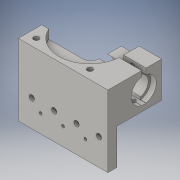
# Autodesk Inventor part: Galvomount-22mm-diameter-Left-Scanlab-V4
Saved by Autodesk Inventor 2016 (Build 200138000, 138)
## iProperties
Created: 2016-08-10
Part Number: Galvomount-22mm-diameter-Left-Scanlab-V4
Material: Generic
Document SubType Name: Modeling
Designer: voigt
Density: 1 g/cm^3
Appearance: Default
Author: voigt
Autodesk Inventor part; units mm, degrees
ref_plane "YZ Plane" through (0, 0, 0) normal (1, 0, 0) x (0, 1, 0)
ref_plane "XZ Plane" through (0, 0, 0) normal (0, 1, 0) x (-1, 0, 0)
ref_plane "XY Plane" through (0, 0, 0) normal (0, 0, 1) x (1, 0, 0)
sketch "Sketch1" plane through (0, 0, 0) normal (0, 0, 1) x (1, 0, 0)
  line L0 (0, 32) -> (0, -52) construction
  line L1 (-60, 0) -> (80, 0) construction
  line L2 (-40, 20) -> (60, 20)
  line L3 (60, 20) -> (60, -40)
  line L4 (60, -40) -> (-40, -40)
  line L5 (-40, -40) -> (-40, 20)
  point P0 (0, 0)
  dimension "d0" = 20
  dimension "d1" = 40
  dimension "d2" = 40
  dimension "d3" = 60
  constraints: 8 end point, 2 parallel, 1 horizontal, 1 perpendicular
  measures "d0" distance between parallel lines of L1 L2
  measures "d1" distance between parallel lines of L4 L1
  measures "d2" distance between parallel lines of L5 L0
  measures "d3" distance between parallel lines of L0 L3
extrude "Extrusion1" add sketch "Sketch1" against normal blind 40
sketch "Sketch2" plane through (0, 0, 0) normal (0, 0, 1) x (1, 0, 0)
  line L0 (-40, 20) -> (60, 20) construction
  line L1 (-40, -40) -> (-40, 20) construction
  line L2 (60, -40) -> (-40, -40) construction
  line L3 (60, 20) -> (60, -40) construction
  line L4 (0, 98) -> (0, -63) construction
  line L5 (-60, 0) -> (80, 0) construction
  line L6 (0, 40) -> (0, 0) construction
  line L7 (-40, 20) -> (60, 20) projected
  line L8 (-35, 40) -> (-35, 0)
  line L9 (35, 0) -> (35, 40)
  arc A0 (35, 40) -> (-35, 40) centre (0, 40) ccw
  arc A1 (-35, 0) -> (35, 0) centre (0, 0) ccw
  point P0 (0, 20)
  dimension "d6" = 70
  constraints: 8 end point, 4 point on circle, 4 tangent, 2 centre point, 2 point on line, 1 midpoint, 1 parallel, 1 perpendicular
  measures "d6" diameter of A1
extrude "Extrusion2" cut sketch "Sketch2" against normal blind 10
sketch "Sketch3" plane through (60, -40, 0) normal (1, 0, 0) x (0, 0, -1)
  line L0 (0, 60) -> (0, 0) construction
  line L1 (0, 0) -> (40, 0) construction
  line L2 (40, 60) -> (40, 0) construction
  line L3 (0, 60) -> (40, 60) construction
  line L4 (0, 40) -> (40, 40) construction
  line L5 (40, 0) -> (40, 60) construction
  line L6 (0, 60) -> (40, 60) construction
  line L7 (20, 60) -> (20, 0) construction
  circle A0 centre (20, 40) radius 11
  dimension "d9" = 22
  constraints: 4 end point, 3 midpoint, 2 point on line, 1 centre point, 1 perpendicular
  measures "d9" diameter of A0
extrude "Extrusion3" cut sketch "Sketch3" against normal up to next
sketch "Sketch6" plane through (0, 0, 0) normal (0, 0, 1) x (1, 0, 0)
  line L0 (0, 44) -> (0, -54) construction
  line L1 (-60, 0) -> (80, 0) construction
  line L2 (-30, 30) -> (30, 30) construction
  line L3 (30, 30) -> (30, -30) construction
  line L4 (30, -30) -> (-30, -30) construction
  line L5 (-30, -30) -> (-30, 30) construction
  point P0 (0, 0)
  dimension "d19" = 60
  dimension "d20" = 60
  constraints: 8 end point, 2 coincident, 2 parallel, 1 horizontal, 1 perpendicular, 2 other
  measures "d19" distance of L2.start L2.end
  measures "d20" distance of L4.end L2.start
hole "Hole1" at (-30, -30, 0) at (30, -30, 0) direction (0, 0, -1) diameter 6 depth 30 tip angle 118
sketch "Sketch16" plane through (-40, -40, 0) normal (-1, 0, 0) x (0, 0, 1)
  line L0 (-40, 0) -> (-40, 60) construction
  line L1 (0, 0) -> (-40, 0) construction
  line L2 (0, 0) -> (0, 60) construction
  line L3 (0, 13) -> (0, 7) construction
  line L4 (-30, 7) -> (-30, 13) construction
  line L5 (-30, 10) -> (0, 10) construction
  circle A0 centre (-20, 40) radius 11 projected
  line L6 (0, 60) -> (-40, 60) projected
  point P0 (0, 40)
  point P1 (-10, 10)
  dimension "d86" = 10
  constraints: 2 end point, 2 midpoint, 1 point on line
  measures "d86" distance from line of L2 point (-10, 10)
hole "Hole7" at (-40, -30, -10) direction (1, 0, 0) diameter 2.156 depth 8.865 tip angle 118 thread size "4-40 UNC" class "2B" standard "ANSI Unified Screw Threads"
sketch "Sketch18" plane through (-40, -40, 0) normal (-1, 0, 0) x (0, 0, 1)
  circle A0 centre (-10, 10) radius 1.078 projected
  line L0 (-40, 0) -> (-40, 60) projected
  line L1 (0, 0) -> (-40, 0) projected
  line L2 (0, 0) -> (0, 60) projected
  circle A1 centre (-20, 40) radius 11 projected
  line L3 (0, 60) -> (-40, 60) projected
  point P0 (0, 40)
extrude "Extrusion10" cut sketch "Sketch18" against normal blind 5 contours A1
sketch "Sketch19" plane through (60, -40, 0) normal (1, 0, 0) x (0, 0, -1)
  line L0 (0, 60) -> (40, 60) projected
  line L1 (0, 60) -> (0, 0) projected
  line L2 (0, 0) -> (40, 0) projected
  line L3 (40, 60) -> (40, 0) projected
  circle A0 centre (20, 40) radius 11 projected
  point P0 (0, 40)
extrude "Extrusion11" cut sketch "Sketch19" against normal blind 6 contours A0
sketch "Sketch23" plane through (60, -40, 0) normal (1, 0, 0) x (0, 0, -1)
  circle A0 centre (20, 40) radius 11 construction
  line L0 (0, 60) -> (0, 0) construction
  line L1 (0, 0) -> (40, 0) construction
  line L2 (40, 60) -> (40, 0) construction
  line L3 (0, 60) -> (40, 60) construction
  line L4 (0, 42.5) -> (34, 42.5)
  line L5 (34, 42.5) -> (34, 37.5)
  line L6 (34, 37.5) -> (0, 37.5)
  line L7 (0, 37.5) -> (0, 42.5)
  line L8 (0, 40) -> (20, 40) construction
  dimension "d119" = 5
  dimension "d120" = 14
  constraints: 10 end point, 2 horizontal, 2 parallel, 1 perpendicular, 1 point on line, 1 other
  measures "d119" distance between parallel lines of L6 L4
  measures "d120" distance from line of L8.end L5
extrude "Extrusion15" cut sketch "Sketch23" against normal up to next
sketch "Sketch24" plane through (-40, 20, -40) normal (0, 1, 0) x (1, 0, 0)
  line L0 (75, -30) -> (75, -40) construction
  line L1 (75, -40) -> (100, -40) construction
  line L2 (100, -40) -> (100, 0) construction
  line L3 (0, 0) -> (100, 0) construction
  line L4 (0, -40) -> (0, 0) construction
  line L5 (0, -40) -> (5, -40) construction
  line L6 (5, -40) -> (5, -30) construction
  line L7 (5, -30) -> (75, -30) construction
  line L8 (100, -6) -> (0, -6) construction
  line L9 (100, -6) -> (0, -6) projected
  line L10 (0, -40) -> (55, -40)
  line L11 (55, -40) -> (55, -6)
  line L12 (55, -6) -> (0, -6)
  line L13 (0, -6) -> (0, -40)
  line L14 (40, -40) -> (40, 0) construction
  line L15 (0, 0) -> (100, 0) construction
  dimension "d123" = 15
  constraints: 10 end point, 2 parallel, 2 perpendicular, 2 point on line, 1 horizontal
  measures "d123" distance between parallel lines of L14 L11
extrude "Extrusion16" cut sketch "Sketch24" against normal blind 34
fillet "Fillet3" radius 10 1 edges at (15, -14, -22)
sketch "Sketch25" plane through (0, 0, -40) normal (0, 0, -1) x (-1, 0, 0)
  line L0 (40, 20) -> (-60, 20) construction
  line L1 (-60, 20) -> (-60, -40) construction
  line L2 (-60, -40) -> (40, -40) construction
  line L3 (40, -40) -> (40, 20) construction
  line L4 (-60, 20) -> (-60, -40) projected
  line L5 (40, -28.922) -> (40, -31.078) projected
  line L6 (-60, -40) -> (40, -40)
  line L7 (40, -40) -> (40, -30)
  line L8 (40, -30) -> (-60, -30)
  line L9 (-60, -30) -> (-60, -40)
  point P0 (0, 0)
  dimension "d127" = 10
  constraints: 8 end point, 2 parallel, 1 horizontal, 1 midpoint, 1 perpendicular
  measures "d127" distance of L7.end L6.end
extrude "Extrusion17" add sketch "Sketch25" along normal blind 40
sketch "Sketch26" plane through (-40, 20, -40) normal (0, 1, 0) x (1, 0, 0)
  line L0 (100, 40) -> (0, 40) construction
  line L1 (55, -6) -> (55, -30) construction
  line L2 (55, -30) -> (75, -30) construction
  line L3 (75, -30) -> (75, -40) construction
  line L4 (75, -40) -> (100, -40) construction
  line L5 (100, -40) -> (100, 0) construction
  line L6 (0, 0) -> (100, 0) construction
  line L7 (0, -6) -> (0, 0) construction
  line L8 (0, -6) -> (55, -6) construction
  line L9 (0, -6) -> (55, -6) projected
  line L10 (0, 0) -> (100, 0) projected
  line L11 (0, -6) -> (55, -6)
  line L12 (55, -6) -> (55, 0)
  line L13 (55, 0) -> (0, 0)
  line L14 (0, 0) -> (0, -6)
  line L15 (55, -6) -> (55, -30) projected
  point P0 (40, -40)
  constraints: 8 end point, 2 parallel, 1 collinear, 1 horizontal, 1 perpendicular, 1 point on line
extrude "Extrusion18" cut sketch "Sketch26" against normal blind 10
sketch "Sketch27" plane through (-40, -30, -40) normal (0, 1, 0) x (1, 0, 0)
  line L0 (100, 0) -> (0, 0) construction
  line L1 (100, 0) -> (100, 40) construction
  line L2 (0, 40) -> (100, 40) construction
  line L3 (0, 0) -> (0, 40) construction
  line L4 (0, -40) -> (0, 40) construction
  line L5 (0, 10) -> (100, 10) construction
  line L6 (40, -40) -> (40, 40) construction
  line L7 (0, 40) -> (100, 40) construction
  point P0 (40, 10)
  point P1 (15, 10)
  point P2 (65, 10)
  point P3 (90, 10)
  dimension "d132" = 10
  dimension "d154" = 25
  dimension "d155" = 25
  dimension "d156" = 25
  constraints: 8 point on line, 4 end point, 1 perpendicular, 1 vertical
  measures "d132" distance between parallel lines of L0 L5
  measures "d154" distance of point (15, 10) point (40, 10)
  measures "d155" distance of point (65, 10) point (40, 10)
  measures "d156" distance of point (65, 10) point (90, 10)
sketch "Sketch28" plane through (60, 20, 0) normal (1, 0, 0) x (0, 0, -1)
  line L0 (34, -22.5) -> (30.7121, -22.5) construction
  arc A0 (9.2879, -22.5) -> (30.7121, -22.5) centre (20, -20) ccw construction
  line L1 (9.2879, -22.5) -> (0, -22.5) construction
  line L2 (0, -22.5) -> (0, -60) construction
  line L3 (0, -60) -> (80, -60) construction
  line L4 (80, -50) -> (80, -60) construction
  line L5 (40, -50) -> (80, -50) construction
  line L6 (40, 0) -> (40, -50) construction
  line L7 (0, 0) -> (40, 0) construction
  line L8 (0, 0) -> (0, -17.5) construction
  line L9 (0, -17.5) -> (9.2879, -17.5) construction
  arc A1 (30.7121, -17.5) -> (9.2879, -17.5) centre (20, -20) ccw construction
  line L10 (30.7121, -17.5) -> (34, -17.5) construction
  line L11 (34, -17.5) -> (34, -22.5) construction
  circle A2 centre (20, -20) radius 14
  point P0 (0, -20)
  dimension "d133" = 28
  constraints: 1 centre point, 1 coincident
  measures "d133" diameter of A2
extrude "Extrusion19" cut sketch "Sketch28" against normal blind 6
sketch "Sketch29" plane through (60, 20, 0) normal (0, 1, 0) x (1, 0, 0)
  line L0 (-6, 6.225) -> (-6, 9.2879) construction
  line L1 (-25.0894, 9.2879) -> (-6, 9.2879) construction
  line L2 (-25.0894, 0) -> (-25.0894, 9.2879) construction
  line L3 (0, 0) -> (-25.0894, 0) construction
  line L4 (0, 6.225) -> (0, 0) construction
  line L5 (0, 6.225) -> (-6, 6.225) construction
  line L6 (-45, 40) -> (-45, 10) construction
  line L7 (-45, 10) -> (-25, 10) construction
  line L8 (-25, 10) -> (-25, 0) construction
  line L9 (-25, 0) -> (0, 0) construction
  line L10 (0, 0) -> (0, 40) construction
  line L11 (-45, 40) -> (0, 40) construction
  point P0 (-60, 0)
  point P1 (-15, 5)
  dimension "d136" = 5
  dimension "d138" = 10
  measures "d136" distance from line of L3 point (-15, 5)
  measures "d138" distance from line of L8 point (-15, 5)
hole "Hole9" at (45, 20, -5) direction (0, -1, 0) diameter 5 end up to surface counterbore diameter 9 counterbore depth 5
sketch "Sketch30" plane through (34.9106, -2.5, 0) normal (0, 1, 0) x (1, 0, 0)
  circle A0 centre (10.0894, 5) radius 4.5 construction
  circle A1 centre (10.0894, 5) radius 2.5 construction
  point P0 (-34.9106, 0)
  constraints: 1 coincident
hole "Hole10" at (45, -2.5, -5) direction (0, -1, 0) diameter 4.134 depth 14.2 tip angle 118 thread size "M5x0.8" class "6H" standard "ISO Metric profile"
hole "Hole11" at (0, -30, -50) at (-25, -30, -50) at (25, -30, -50) at (50, -30, -50) direction (0, -1, 0) diameter 6 end through all counterbore diameter 10.5 counterbore depth 6.5
sketch "Sketch31" plane through (0, 0, -40) normal (0, 0, -1) x (-1, 0, 0)
  line L0 (-15, 10) -> (-15, 20) construction
  line L1 (-15, 20) -> (-60, 20) construction
  line L2 (-60, 20) -> (-60, -30) construction
  line L3 (-60, -30) -> (40, -30) construction
  line L4 (40, -30) -> (40, 10) construction
  line L5 (40, 10) -> (-15, 10) construction
  line L6 (-60, -10) -> (40, -10) construction
  point P0 (0, 0)
  point P1 (-35, -10)
  point P2 (15, -10)
  point P3 (-10, -10)
  dimension "d164" = 20
  dimension "d165" = 25
  dimension "d166" = 25
  constraints: 3 point on line, 2 end point, 2 midpoint, 1 perpendicular
  measures "d164" distance between parallel lines of L5 L6
  measures "d165" distance of point (-10, -10) point (15, -10)
  measures "d166" distance of point (-10, -10) point (-35, -10)
hole "Hole12" at (35, -10, -40) at (-15, -10, -40) at (10, -10, -40) direction (0, 0, 1) diameter 3.242 depth 10 tip angle 118 thread size "M4x0.7" class "6H" standard "ANSI Metric M Profile"
sketch "Sketch32" plane through (-40, -30, -40) normal (0, 1, 0) x (1, 0, 0)
  circle A0 centre (65, 10) radius 5.25 construction
  circle A1 centre (40, 10) radius 5.25 construction
  circle A2 centre (15, 10) radius 5.25 construction
  circle A3 centre (90, 10) radius 5.25 construction
  line L0 (100, 0) -> (0, 0) construction
  line L1 (100, 0) -> (100, 40) construction
  line L2 (0, 40) -> (100, 40) construction
  line L3 (0, 0) -> (0, 40) construction
  line L4 (100, 0) -> (100, 40) construction
  line L5 (100, 20) -> (0, 20) construction
  line L6 (0, 0) -> (0, 40) construction
  point P0 (40, -40)
  point P1 (50, 20)
  point P2 (25, 20)
  point P3 (75, 20)
  dimension "d174" = 50
  dimension "d175" = 25
  dimension "d176" = 25
  constraints: 3 midpoint, 2 end point, 2 point on line
  measures "d174" distance from line of L3 point (50, 20)
  measures "d175" distance from line of L3 point (25, 20)
  measures "d176" distance of point (50, 20) point (75, 20)
hole "Hole13" at (10, -30, -60) at (-15, -30, -60) at (35, -30, -60) direction (0, -1, 0) diameter 3.242 end through all thread size "M4x0.7" class "6H" standard "ANSI Metric M Profile"
body "Solid1"
